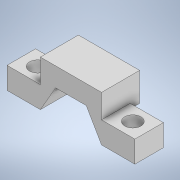
# Autodesk Inventor part: shell 1.0 screw top
Saved by Autodesk Inventor 2020.2 (Build 242310000, 310)
## iProperties
Created: 2020-02-28
Part Number: shell 1.0 screw top
Material: Generic
Document SubType Name: Modeling
Designer: ColinP
Density: 1 g/cm^3
Appearance: Default
Author: ColinP
Autodesk Inventor part; units mm, degrees
ref_plane "YZ Plane" through (0, 0, 0) normal (1, 0, 0) x (0, 1, 0)
ref_plane "XZ Plane" through (0, 0, 0) normal (0, 1, 0) x (-1, 0, 0)
ref_plane "XY Plane" through (0, 0, 0) normal (0, 0, 1) x (1, 0, 0)
sketch "Sketch1" plane through (0, 0, 0) normal (0, 0, 1) x (1, 0, 0)
  line L0 (0, 0) -> (-6.4135, 0)
  line L1 (-6.4135, 0) -> (-3.2004, 5.5653)
  line L2 (-3.2004, 5.5653) -> (3.2258, 5.5653)
  line L3 (3.2258, 5.5653) -> (6.4389, 0)
  line L4 (6.4389, 0) -> (3.2258, -5.5653)
  line L5 (3.2258, -5.5653) -> (-3.2004, -5.5653)
  line L6 (-3.2004, -5.5653) -> (-6.4135, 0)
  line L7 (-6.4135, 0) -> (-13.4135, 0)
  line L8 (-6.4135, 0) -> (0.5865, 0) construction
  line L9 (-13.4135, 0) -> (-13.4135, 5.5653)
  line L10 (-13.4135, 5.5653) -> (-13.4135, 9.5653)
  line L11 (-13.4135, 9.5653) -> (13.4389, 9.5653)
  line L12 (13.4389, 9.5653) -> (13.4389, 0)
  line L13 (13.4389, 0) -> (6.4389, 0)
  line L14 (13.4389, 9.5653) -> (13.4389, 4.5653)
  line L15 (13.4389, 4.5653) -> (6.4389, 4.5653)
  line L16 (6.4389, 4.5653) -> (6.4389, 9.5653)
  line L17 (-13.4135, 9.5653) -> (-6.4135, 9.5653)
  line L18 (-6.4135, 9.5653) -> (-6.4135, 4.5653)
  line L19 (-6.4135, 4.5653) -> (-13.4135, 4.5653)
  dimension "d0" = 6.4135
  dimension "d1" = 6.4262
  dimension "d2" = 60
  dimension "d3" = 6.4262
  dimension "d4" = 120
  dimension "d5" = 6.4262
  dimension "d6" = 120
  dimension "d7" = 6.4262
  dimension "d8" = 120
  dimension "d9" = 6.4262
  dimension "d10" = 120
  dimension "d11" = 7
  dimension "d12" = 180
  dimension "d13" = 4
  dimension "d15" = 5
  dimension "d16" = 7
  dimension "d17" = 7
  dimension "d20" = 7
  constraints: 40 end point, 8 point on line, 6 perpendicular, 3 horizontal, 3 parallel, 1 collinear
  measures "d0" distance of L0.start L0.end
  measures "d1" distance of L0.end L1.end
  measures "d2" angle of L0 L1
  measures "d3" distance of L1.end L2.end
  measures "d4" angle of L1 L2
  measures "d5" distance of L2.end L3.end
  measures "d6" angle of L2 L3
  measures "d7" distance of L3.end L4.end
  measures "d8" angle of L3 L4
  measures "d9" distance of L4.end L5.end
  measures "d10" angle of L4 L5
  measures "d11" distance of L0.end L7.end
  measures "d12" angle of L7 L8
  measures "d13" distance of L9.end L10.end
  measures "d15" distance of L11.end L14.end
  measures "d16" distance of L14.end L15.end
  measures "d17" distance of L10.end L17.end
  measures "d20" distance of L12.end L3.end
extrude "Extrusion1" add sketch "Sketch1" along normal blind 6 contours L7 L9 L19 L18 L11 L16 L15 L12 L13 L3 L2 L1
sketch "Sketch3" plane through (0, 0, 0) normal (0, 0, -1) x (-1, 0, 0)
  line L0 (-6.4389, 4.5653) -> (-6.4389, 9.5653) projected
  line L1 (-6.4389, 9.5653) -> (-6.4389, 3.5653)
  line L2 (-6.4389, 3.5653) -> (6.4135, 3.5653)
  line L3 (6.4135, 9.5653) -> (6.4135, 4.5653) projected
  line L4 (-6.4389, 9.5653) -> (6.4135, 9.5653) projected
  line L5 (6.4135, 3.5653) -> (6.4135, 9.5653)
  line L6 (6.4135, 9.5653) -> (-6.4389, 9.5653)
  point P0 (0, 0)
  point P1 (6.4135, 4.5653)
  point P2 (-6.4389, 4.5653)
  dimension "d30" = 6
  constraints: 8 end point, 3 perpendicular, 1 collinear
  measures "d30" distance of L0.end L1.end
extrude "Extrusion2" add sketch "Sketch3" along normal blind 2
sketch "Sketch4" plane through (-13.4135, 0, 0) normal (0, -1, 0) x (1, 0, 0)
  line L0 (0, 0) -> (0, 6) projected
  line L1 (0, 3) -> (26.8524, 3)
  line L2 (26.8524, 0) -> (26.8524, 6) projected
  line L3 (13.4262, 3) -> (3.4262, 3)
  line L4 (3.4262, 3) -> (23.4262, 3)
  point P0 (13.4135, 0)
  dimension "d36" = 10
  dimension "d37" = 20
  dimension "d38" = 0
  constraints: 6 end point, 3 midpoint, 1 collinear, 1 point on line
  measures "d36" distance of L3.start L3.end
  measures "d37" distance of L3.end L4.end
  measures "d38" distance between parallel lines of L4 L3
hole "Hole2" at (-9.9873, 0, 3) at (10.0127, 0, 3) direction (0, 1, 0) diameter 3.4 end through all clearance for "Flat Head Machine Screw" size "M3" standard "Ansi Metric M Profile"
body "Solid1"
